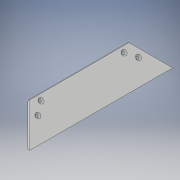
# Autodesk Inventor part: Tyl2
Saved by Autodesk Inventor 2019 (Build 230136000, 136)
## iProperties
Created: 2021-12-11
Part Number: Tyl2
Material: Ogólny
Document SubType Name: Modeling
Designer: Michał
Density: 1 g/cm^3
Appearance: Domyślna
Author: Michał
Autodesk Inventor part; units mm, degrees
ref_plane "YZ Plane" through (0, 0, 0) normal (1, 0, 0) x (0, 1, 0)
ref_plane "XZ Plane" through (0, 0, 0) normal (0, 1, 0) x (-1, 0, 0)
ref_plane "XY Plane" through (0, 0, 0) normal (0, 0, 1) x (1, 0, 0)
sketch "Szkic1" plane through (0, 0, 0) normal (0, 0, 1) x (1, 0, 0)
  line L0 (0, 0) -> (2.8284, 0)
  line L1 (2.8284, 0) -> (-27.1716, 30)
  line L2 (-27.1716, 30) -> (-27.1716, 27.1716)
  line L3 (-27.1716, 27.1716) -> (0, 0)
  line L4 (-27.1716, 30) -> (-28, 30)
  line L5 (-28, 30) -> (-28, 28)
  line L6 (-28, 28) -> (-27.1716, 28)
  line L7 (-27.1716, 28) -> (-27.1716, 30)
  line L8 (-28, 28) -> (-27.1716, 27.1716)
  dimension "d1" = 30
  dimension "d3" = 45
  dimension "d20" = 2
  dimension "d21" = 2
  constraints: 18 end point, 3 parallel, 2 horizontal, 2 perpendicular, 1 collinear
  measures "d1" distance from line of L0 L1.end
  measures "d3" angle of L0 L3
  measures "d20" distance between parallel lines of L1 L3
  measures "d21" distance of L4.end L5.end
extrude "Wyciągnięcie proste1" add sketch "Szkic1" along normal blind 196.178
sketch "Szkic4" plane through (-28, 28, 0) normal (-1, 0, 0) x (0, 0, 1)
  line L0 (0, 0) -> (0, -28) projected
  line L1 (0, 2) -> (196.178, 2) projected
  line L2 (0, -28) -> (0, 2)
  line L3 (0, 2) -> (30, 2)
  line L4 (30, 2) -> (0, -28)
  line L5 (98.089, 2) -> (98.089, -28) construction
  line L6 (196.178, 0) -> (196.178, -28)
  line L7 (196.178, -28) -> (196.178, 2)
  line L8 (196.178, 2) -> (166.178, 2)
  line L9 (166.178, 2) -> (196.178, -28)
  dimension "d22" = 45
  constraints: 16 end point, 3 symmetric about line, 2 perpendicular, 1 midpoint, 1 vertical
  measures "d22" angle of L0 L4
extrude "Wyciągnięcie proste3" cut sketch "Szkic4" against normal through all
sketch "Szkic5" plane through (2.8284, 0, 0) normal (0.7071, 0.7071, 0) x (-0.7071, 0.7071, 0)
  line L0 (41.598, 28) -> (41.598, 168.178) construction
  line L1 (41.598, 98.089) -> (0, 98.089) construction
  line L2 (0, 0) -> (0, 196.178) construction
  point P0 (2, 0)
  point P1 (36.298, 155.089)
  point P2 (36.298, 41.089)
  point P3 (25.298, 167.089)
  point P4 (25.298, 29.089)
  dimension "d25" = 57
  dimension "d26" = 5.3
  dimension "d34" = 69
  dimension "d35" = 16.3
  constraints: 2 end point, 2 midpoint, 2 symmetric about line
  measures "d25" distance from line of L1 point (36.298, 155.089)
  measures "d26" distance from line of L0 point (36.298, 155.089)
  measures "d34" distance from line of L1 point (25.298, 167.089)
  measures "d35" distance from line of L0 point (25.298, 167.089)
hole "Otwór2" at (-22.8381, 25.6665, 155.089) at (-22.8381, 25.6665, 41.089) at (-15.0599, 17.8884, 167.089) at (-15.0599, 17.8884, 29.089) direction (-0.7071, -0.7071, 0) diameter 3.2 end through all countersink diameter 6.9 countersink angle 84.225 clearance for "Śruba ze łbem stożkowym ISO 2009/7046" size "M3" standard "ISO"
